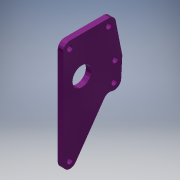
# Autodesk Inventor part: carriage plate for intake
Saved by Autodesk Inventor 2017 SP1 (Build 210196100, 196)
## iProperties
Created: 2018-01-19
Part Number: carriage plate for intake
Material: Aluminum 6061
Document SubType Name: Modeling
Designer: Ben
Density: 2.7 g/cm^3
Appearance: Smooth - Purple
Mass: 147.998 g
Surface Area: 209.147 cm^2
Volume: 54.8139 cm^3
Author: Ben
Autodesk Inventor part; units mm, degrees
ref_plane "YZ Plane" through (0, 0, 0) normal (1, 0, 0) x (0, 1, 0)
ref_plane "XZ Plane" through (0, 0, 0) normal (0, 1, 0) x (-1, 0, 0)
ref_plane "XY Plane" through (0, 0, 0) normal (0, 0, 1) x (1, 0, 0)
sketch "Sketch1" plane through (0, 0, 0) normal (1, 0, 0) x (0, 1, 0)
  line L0 (-162.6843, 12.7) -> (420.7488, 12.7) construction
  line L1 (420.7488, 12.7) -> (420.7488, -12.7) construction
  line L2 (420.7488, -12.7) -> (-162.6843, -12.7) construction
  line L3 (-162.6843, -12.7) -> (-162.6843, 12.7) construction
  line L4 (0, 0) -> (0, -26.6192) construction
  circle A0 centre (0, -26.6192) radius 3.302
  circle A1 centre (38.1, 26.6192) radius 2.54
  circle A2 centre (-76.2, 26.6192) radius 2.54
  line L5 (38.1, 26.6192) -> (-76.2, 26.6192) construction
  line L6 (0, 0) -> (0, 26.6192) construction
  circle A3 centre (0, -26.6192) radius 15.875 construction
  circle A4 centre (38.1, 26.6192) radius 15.875 construction
  circle A5 centre (-76.2, 26.6192) radius 15.875 construction
  line L7 (0, -26.6192) -> (-76.2, 26.6192) construction
  arc A6 (46.1645, 26.6192) -> (38.1, 34.6837) centre (38.1, 26.6192) ccw
  line L8 (38.1, 34.6837) -> (-76.2, 34.6837)
  line L9 (46.1645, 26.6192) -> (46.1645, -19.05)
  line L10 (-76.2, 26.6192) -> (-76.2, 0) construction
  line L11 (38.1, 26.6192) -> (38.1, 0) construction
  line L12 (46.1645, 0) -> (-87.2704, 0) construction
  line L13 (0, -26.6192) -> (38.1, 26.6192) construction
  line L14 (0, -26.6192) -> (0, -52.0192) construction
  line L15 (13.9446, -26.6192) -> (-16.4809, -26.6192) construction
  circle A7 centre (38.1, -19.05) radius 2.54
  line L16 (38.1, -19.05) -> (38.1, 0) construction
  arc A8 (39.6714, -26.9599) -> (46.1645, -19.05) centre (38.1, -19.05) ccw
  arc A9 (-29.845, -22.7596) -> (-22.6667, -33.4524) centre (-22.225, -25.4) ccw
  line L17 (-22.225, -12.7) -> (-22.225, -25.4) construction
  circle A10 centre (-22.225, -25.4) radius 2.54
  arc A11 (-0.4417, -34.6716) -> (1.5714, -34.5291) centre (0, -26.6192) ccw
  line L18 (39.6714, -26.9599) -> (1.5714, -34.5291)
  line L19 (-0.4417, -34.6716) -> (-22.6667, -33.4524)
  circle A12 centre (2.8575, 12.7) radius 11.1125
  arc A13 (-76.2, 34.6837) -> (-80.8188, 20.0084) centre (-76.2, 26.6192) ccw
  line L20 (-65.9165, 81.474) -> (15.5575, 0) construction
  line L21 (-80.8188, 20.0084) -> (-32.8463, -13.5084)
  arc A14 (-29.845, -22.7596) -> (-32.8463, -13.5084) centre (-37.465, -20.1193) ccw
  point P0 (0, -42.4942)
  point P1 (-162.6843, 0)
  dimension "d3" = 31.75
  dimension "d0" = 25.4
  dimension "d1" = 6.604
  dimension "d2" = 13.9192
  dimension "d4" = 38.1
  dimension "d5" = 76.2
  dimension "d10" = 25.4
  dimension "d14" = 6.35
  dimension "d22" = 12.7
  dimension "d32" = 22.225
  dimension "d33" = 22.225
  dimension "d47" = 0
  dimension "d49" = 45
  dimension "d50" = 30.607
  dimension "d52" = 35.2425
  dimension "d55" = 5.08
  dimension "d57" = 4.7625
  constraints: 44 end point, 14 centre point, 13 point on circle, 12 coincident, 11 point on line, 11 tangent, 6 equal radius, 6 vertical, 5 horizontal, 3 parallel, 3 perpendicular, 1 collinear, 1 midpoint, 1 vertical alignment, 4 other
  measures "d0" distance of L0.end L1.end
  measures "d1" diameter of A0
  measures "d2" distance from line of L2 L4.end
  measures "d4" horizontal distance of L5.start L4.end
  measures "d5" distance from line of A2.centre L6
  measures "d10" distance of L13.start L14.end
  measures "d14" distance from line of L2 L16.start
  measures "d22" distance of L17.start L17.end
  measures "d32" distance between parallel lines of L4 L17
  measures "d33" diameter of A12
  measures "d47" distance from line of A12.centre L0
  measures "d49" angle of L20 L12
  measures "d50" distance from line of L9 L20.end
  measures "d52" horizontal distance of L16.start A12.centre
  measures "d55" diameter of A1
  measures "d57" radial gap between concentric circles of A0 A11
extrude "Extrusion1" add sketch "Sketch1" along normal blind 6.35
body "Solid1"
